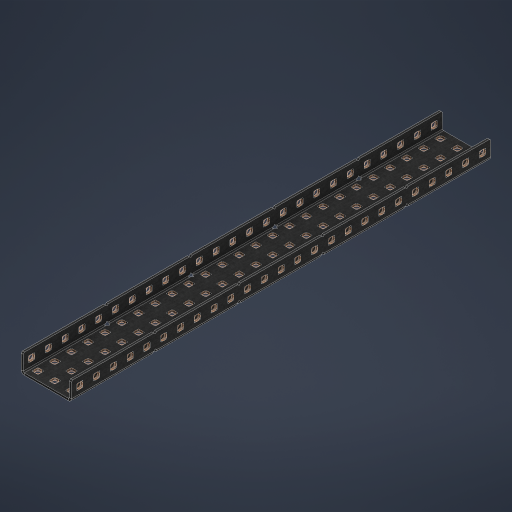
# Autodesk Inventor part: Alu C 1x3x1x35
Saved by Autodesk Inventor 2024 (Build 280153000, 153)
## iProperties
Created: 2022-07-28
Part Number: Alu C 1x3x1x35
Material: Generic
Document SubType Name: Sheet Metal
Designer: ylu12
Density: 1 g/cm^3
Sheet Metal Rule: Default
Appearance: Aluminum
Author: ylu12
Autodesk Inventor part; units mm, degrees
ref_plane "YZ Plane" through (0, 0, 0) normal (1, 0, 0) x (0, 1, 0)
ref_plane "XZ Plane" through (0, 0, 0) normal (0, 1, 0) x (-1, 0, 0)
ref_plane "XY Plane" through (0, 0, 0) normal (0, 0, 1) x (1, 0, 0)
sketch "Sketch1" plane through (0, 0, 0) normal (0, 1, 0) x (-1, 0, 0)
  line L0 (-19.05, 0) -> (19.05, 0)
  line L1 (19.05, 0) -> (19.05, -317.5)
  line L2 (19.05, -317.5) -> (-19.05, -317.5)
  line L3 (-19.05, -317.5) -> (-19.05, 0)
  line L4 (19.05, 0) -> (-19.05, -317.5) construction
  point P0 (0, 0)
  point P1 (0, 0)
  dimension "d0" = 38.1
  dimension "d1" = 317.5
  constraints: 10 end point, 2 parallel, 1 coincident, 1 horizontal, 1 midpoint, 1 perpendicular
  measures "d0" distance of L1.end L2.end
  measures "d1" distance of L0.end L1.end
extrude "Plate1" add sketch "Sketch1" along normal blind 1.5875
sketch "Sketch2" plane through (17.4625, 0, -317.5) normal (1, 0, 0) x (0, 1, 0)
  line L0 (0, 317.5) -> (0, 0)
  line L1 (0, 0) -> (14.2875, 0)
  line L2 (14.2875, 0) -> (14.2875, 317.5)
  line L3 (14.2875, 317.5) -> (0, 317.5)
  constraints: 6 end point, 1 horizontal, 1 perpendicular, 1 vertical
edge flange "Flanges" height 12.7 angle 90 thickness 1.5875 bend radius 0.7937 thickness toward (1, 0, 0) relief straight relief width 1.5875 relief depth 0.7937 corner gap 1.5875 corner form 0 edges at (19.05, 1.5875, -158.75) (-19.05, 1.5875, -158.75) wall of the first edge with corners at (17.4625, 0, 0) (17.4625, 0, -317.5) (17.4625, 14.2875, -317.5) (17.4625, 14.2875, 0)
bend "Bend1"
corner "Corner1"
sketch "Sketch3" plane through (19.05, 2.3812, -317.5) normal (1, 0, 0) x (0, 0, -1)
  line L0 (-312.9534, 7.8677) -> (-309.3466, 7.8677)
  line L1 (-308.8386, 7.3597) -> (-308.8386, 3.7529)
  line L2 (-309.3466, 3.2449) -> (-312.9534, 3.2449)
  line L3 (-313.4614, 3.7529) -> (-313.4614, 7.3597)
  arc A0 (-312.9534, 7.8677) -> (-313.4614, 7.3597) centre (-312.9534, 7.3597) ccw
  arc A1 (-308.8386, 7.3597) -> (-309.3466, 7.8677) centre (-309.3466, 7.3597) ccw
  arc A2 (-309.3466, 3.2449) -> (-308.8386, 3.7529) centre (-309.3466, 3.7529) ccw
  arc A3 (-313.4614, 3.7529) -> (-312.9534, 3.2449) centre (-312.9534, 3.7529) ccw
  line L4 (-317.5, 0) -> (-317.5, 11.9062) construction
  line L5 (-317.5, 11.9062) -> (0, 11.9062) construction
  line L6 (-312.9534, 7.3597) -> (-309.3466, 3.7529) construction
  point P0 (-317.5, -2.3813)
  point P1 (-308.8386, 3.2449)
  point P2 (-313.4614, 3.2449)
  point P3 (-311.15, 5.5563)
  dimension "d16" = 4.6228
  dimension "d17" = 0.508
  dimension "d20" = 6.35
  dimension "d21" = 6.35
  constraints: 10 end point, 8 point on circle, 8 tangent, 4 centre point, 4 point on line, 3 equal radius, 2 parallel, 2 perpendicular, 1 horizontal, 1 midpoint
  measures "d16" distance of point (-308.839, 3.245) point (-313.461, 3.245)
  measures "d17" radius of A0
  measures "d20" distance from line of point (-311.15, 5.556) L4
  measures "d21" distance from line of L5 point (-311.15, 5.556)
extrude "Flange Stamp" cut sketch "Sketch3" against normal blind 1.5875
sketch "Sketch7" plane through (19.05, 2.3812, 0) normal (1, 0, 0) x (0, 0, -1)
  arc A0 (4.5466, 7.8677) -> (4.0386, 7.3597) centre (4.5466, 7.3597) ccw construction
  arc A1 (8.1534, 3.2449) -> (8.6614, 3.7529) centre (8.1534, 3.7529) ccw construction
  circle A2 centre (6.35, 5.5563) radius 2.1844
  line L0 (4.5466, 7.3597) -> (8.1534, 3.7529) construction
  point P0 (0, -2.3813)
  dimension "d46" = 4.3688
  constraints: 2 end point, 1 centre point, 1 midpoint
  measures "d46" diameter of A2
surface extrude "Flange Circle" sketch "Sketch7" against normal up to surface (1.5875 mm away) shown yes curves A2
ref_plane "Flange Pattern Plane" through (19.05, 7.9375, -4.5466) normal (0, 1, 0) x (1, 0, 0)
pattern_sketch "Flange Pattern" of "Flange Circle", "Flange Stamp" from (19.05, 7.9375, -6.35) facing (1, 0, 0) copies at (19.05, 7.9375, -19.05) facing (1, 0, 0) at (19.05, 7.9375, -31.75) facing (1, 0, 0) at (19.05, 7.9375, -44.45) facing (1, 0, 0) at (19.05, 7.9375, -57.15) facing (1, 0, 0) at (19.05, 7.9375, -69.85) facing (1, 0, 0) at (-19.05, 7.9375, -6.35) facing (-1, 0, 0) at (-19.05, 7.9375, -19.05) facing (-1, 0, 0) at (-19.05, 7.9375, -31.75) facing (-1, 0, 0) at (-19.05, 7.9375, -44.45) facing (-1, 0, 0) at (-19.05, 7.9375, -57.15) facing (-1, 0, 0) at (-19.05, 7.9375, -69.85) facing (-1, 0, 0) at (19.05, 7.9375, -82.55) facing (1, 0, 0) at (-19.05, 7.9375, -82.55) facing (-1, 0, 0) at (19.05, 7.9375, -95.25) facing (1, 0, 0) at (-19.05, 7.9375, -95.25) facing (-1, 0, 0) at (19.05, 7.9375, -107.95) facing (1, 0, 0) at (-19.05, 7.9375, -107.95) facing (-1, 0, 0) at (19.05, 7.9375, -120.65) facing (1, 0, 0) at (-19.05, 7.9375, -120.65) facing (-1, 0, 0) at (19.05, 7.9375, -133.35) facing (1, 0, 0) at (-19.05, 7.9375, -133.35) facing (-1, 0, 0) at (19.05, 7.9375, -146.05) facing (1, 0, 0) at (-19.05, 7.9375, -146.05) facing (-1, 0, 0) at (19.05, 7.9375, -158.75) facing (1, 0, 0) at (-19.05, 7.9375, -158.75) facing (-1, 0, 0) at (19.05, 7.9375, -171.45) facing (1, 0, 0) at (-19.05, 7.9375, -171.45) facing (-1, 0, 0) at (19.05, 7.9375, -184.15) facing (1, 0, 0) at (-19.05, 7.9375, -184.15) facing (-1, 0, 0) at (19.05, 7.9375, -196.85) facing (1, 0, 0) at (-19.05, 7.9375, -196.85) facing (-1, 0, 0) at (19.05, 7.9375, -209.55) facing (1, 0, 0) at (-19.05, 7.9375, -209.55) facing (-1, 0, 0) at (19.05, 7.9375, -222.25) facing (1, 0, 0) at (-19.05, 7.9375, -222.25) facing (-1, 0, 0) at (19.05, 7.9375, -234.95) facing (1, 0, 0) at (-19.05, 7.9375, -234.95) facing (-1, 0, 0) at (19.05, 7.9375, -247.65) facing (1, 0, 0) at (-19.05, 7.9375, -247.65) facing (-1, 0, 0) at (19.05, 7.9375, -260.35) facing (1, 0, 0) at (-19.05, 7.9375, -260.35) facing (-1, 0, 0) at (19.05, 7.9375, -273.05) facing (1, 0, 0) at (-19.05, 7.9375, -273.05) facing (-1, 0, 0) at (19.05, 7.9375, -285.75) facing (1, 0, 0) at (-19.05, 7.9375, -285.75) facing (-1, 0, 0) at (19.05, 7.9375, -298.45) facing (1, 0, 0) at (-19.05, 7.9375, -298.45) facing (-1, 0, 0) at (19.05, 7.9375, -311.15) facing (1, 0, 0) at (-19.05, 7.9375, -311.15) facing (-1, 0, 0)
sketch "Sketch8" plane through (0, 0, 0) normal (0, -1, 0) x (1, 0, 0)
  line L0 (16.6687, 0) -> (-16.6687, 0) construction
  line L1 (14.5034, -4.0386) -> (10.8966, -4.0386)
  line L2 (10.3886, -4.5466) -> (10.3886, -8.1534)
  line L3 (10.8966, -8.6614) -> (14.5034, -8.6614)
  line L4 (15.0114, -8.1534) -> (15.0114, -4.5466)
  arc A0 (15.0114, -4.5466) -> (14.5034, -4.0386) centre (14.5034, -4.5466) ccw
  arc A1 (14.5034, -8.6614) -> (15.0114, -8.1534) centre (14.5034, -8.1534) ccw
  arc A2 (10.3886, -8.1534) -> (10.8966, -8.6614) centre (10.8966, -8.1534) ccw
  arc A3 (10.8966, -4.0386) -> (10.3886, -4.5466) centre (10.8966, -4.5466) ccw
  line L5 (14.5034, -4.5466) -> (10.8966, -8.1534) construction
  line L6 (19.05, 0) -> (19.05, -317.5) construction
  point P0 (0, 0)
  point P1 (10.3886, -8.6614)
  point P2 (15.0114, -8.6614)
  point P3 (12.7, -6.35)
  dimension "d49" = 4.6228
  dimension "d50" = 0.508
  dimension "d51" = 6.35
  dimension "d52" = 6.35
  constraints: 10 end point, 8 point on circle, 8 tangent, 4 centre point, 4 point on line, 3 equal radius, 2 parallel, 2 perpendicular, 1 horizontal, 1 midpoint
  measures "d49" distance of point (15.011, -8.661) point (10.389, -8.661)
  measures "d50" radius of A0
  measures "d51" distance from line of L6 point (12.7, -6.35)
  measures "d52" distance from line of L0 point (12.7, -6.35)
extrude "Body Stamp" cut sketch "Sketch8" against normal blind 1.5875
sketch "Sketch9" plane through (0, 0, 0) normal (0, -1, 0) x (1, 0, 0)
  arc A0 (15.0114, -4.5466) -> (14.5034, -4.0386) centre (14.5034, -4.5466) ccw construction
  arc A1 (10.3886, -8.1534) -> (10.8966, -8.6614) centre (10.8966, -8.1534) ccw construction
  line L0 (14.5034, -4.5466) -> (10.8966, -8.1534) construction
  circle A2 centre (12.7, -6.35) radius 2.1844
  point P0 (0, 0)
  dimension "d55" = 4.3688
  constraints: 2 end point, 1 centre point, 1 midpoint
  measures "d55" diameter of A2
surface extrude "Body Circle" sketch "Sketch9" against normal up to surface (1.5875 mm away) shown yes curves A2
pattern_sketch "Body Pattern" of "Body Stamp", "Body Circle" from (12.7, 0, -6.35) copies at (12.7, 0, -19.05) at (12.7, 0, -31.75) at (12.7, 0, -44.45) at (12.7, 0, -57.15) at (12.7, 0, -69.85) at (12.7, 0, -82.55) at (12.7, 0, -95.25) at (12.7, 0, -107.95) at (12.7, 0, -120.65) at (12.7, 0, -133.35) at (12.7, 0, -146.05) at (12.7, 0, -158.75) at (12.7, 0, -171.45) at (12.7, 0, -184.15) at (12.7, 0, -196.85) at (12.7, 0, -209.55) at (12.7, 0, -222.25) at (12.7, 0, -234.95) at (12.7, 0, -247.65) at (12.7, 0, -260.35) at (12.7, 0, -273.05) at (12.7, 0, -285.75) at (12.7, 0, -298.45) at (12.7, 0, -311.15) at (0, 0, -6.35) at (0, 0, -19.05) at (0, 0, -31.75) at (0, 0, -44.45) at (0, 0, -57.15) at (0, 0, -69.85) at (0, 0, -82.55) at (0, 0, -95.25) at (0, 0, -107.95) at (0, 0, -120.65) at (0, 0, -133.35) at (0, 0, -146.05) at (0, 0, -158.75) at (0, 0, -171.45) at (0, 0, -184.15) at (0, 0, -196.85) at (0, 0, -209.55) at (0, 0, -222.25) at (0, 0, -234.95) at (0, 0, -247.65) at (0, 0, -260.35) at (0, 0, -273.05) at (0, 0, -285.75) at (0, 0, -298.45) at (0, 0, -311.15) at (-12.7, 0, -6.35) at (-12.7, 0, -19.05) at (-12.7, 0, -31.75) at (-12.7, 0, -44.45) at (-12.7, 0, -57.15) at (-12.7, 0, -69.85) at (-12.7, 0, -82.55) at (-12.7, 0, -95.25) at (-12.7, 0, -107.95) at (-12.7, 0, -120.65) at (-12.7, 0, -133.35) at (-12.7, 0, -146.05) at (-12.7, 0, -158.75) at (-12.7, 0, -171.45) at (-12.7, 0, -184.15) at (-12.7, 0, -196.85) at (-12.7, 0, -209.55) at (-12.7, 0, -222.25) at (-12.7, 0, -234.95) at (-12.7, 0, -247.65) at (-12.7, 0, -260.35) at (-12.7, 0, -273.05) at (-12.7, 0, -285.75) at (-12.7, 0, -298.45) at (-12.7, 0, -311.15)
sketch "Arc Length" plane through (17.4625, 2.3812, 0) normal (0, 0, 1) x (1, 0, 0)
  line L0 (0, 0) -> (1.5875, 0) construction
  arc A0 (-0.7937, -0.7937) -> (0, 0) centre (-0.7937, 0) ccw construction
  line L1 (-0.7937, -2.3812) -> (-0.7937, -0.7937) construction
  arc A1 (-0.7937, -2.3812) -> (1.5875, 0) centre (-0.7937, 0) ccw construction
  point P0 (-17.4625, -2.3812)
  dimension "d85" = 3.7405
  dimension "d92" = 1.2468
sketch "Sketch13" plane through (19.05, 14.2875, 0) normal (1, 0, 0) x (0, 0, -1)
  line L0 (0, 0) -> (317.5, 0) construction
  line L1 (62.4078, 0) -> (63.4238, -1.016)
  line L2 (63.4238, -1.016) -> (64.4398, 0)
  line L3 (62.4078, 0) -> (64.4398, 0)
  line L4 (317.5, -11.9062) -> (0, -11.9062) construction
  line L5 (63.4238, -10.8903) -> (61.161, -13.1531)
  line L6 (61.161, -13.1531) -> (63.4238, -15.4159)
  line L7 (63.4238, -15.4159) -> (65.6866, -13.1531)
  line L8 (65.6866, -13.1531) -> (63.4238, -10.8903)
  line L9 (63.4238, -10.8903) -> (63.4238, -15.4159) construction
  line L10 (63.4238, -1.016) -> (63.4238, -10.8903) construction
  line L11 (0, -11.9062) -> (317.5, -11.9062) construction
  point P0 (0, -14.2875)
  dimension "d86" = 4.5256
  dimension "d88" = 1.016
  dimension "d91" = 1.016
  dimension "d102" = 63.4238
  constraints: 19 end point, 6 perpendicular, 2 point on line, 2 vertical, 1 collinear
  measures "d86" distance of L5.start L6.end
  measures "d88" distance from line of L0 L1.end
  measures "d91" distance from line of L5.start L11
  measures "d102" distance from line of L0.start L10
cut across bends "Notch" sketch "Sketch13" k factor 0.44
mirror "Notch Mirror" about plane through (0, 0, 0) normal (1, 0, 0) of "Notch"
pattern_linear "Notch Pattern" count 4 spacing 63.5 along (0, 0, -1) of "Notch", "Notch Mirror"
chamfer "End Chamfer" distance 1.016 angle 45 4 edges at (-18.2562, 14.2875, 0) (18.2562, 14.2875, 0) (-18.2562, 14.2875, -317.5) (18.2563, 14.2875, -317.5)
sketch "Sketch14" plane through (-19.05, 2.3813, 127) normal (1, 0, 0) x (0, 0, -1)
  line L0 (127, 11.9063) -> (444.5, 11.9063) construction
  line L1 (127, 0) -> (127, 11.9063) construction
  line L2 (127, -2.3813) -> (444.5, -2.3813) construction
  line L3 (127, 11.9063) -> (444.5, 11.9063)
  line L4 (444.5, 11.9063) -> (444.5, -2.3813)
  line L5 (444.5, -2.3813) -> (127, -2.3813)
  line L6 (127, -2.3813) -> (127, 11.9063)
  point P0 (127, -2.3812)
  point P1 (382.0521, -1.9844)
  constraints: 8 end point, 2 collinear, 2 parallel, 1 horizontal, 1 perpendicular, 1 other
extrude "Half Cut" [suppressed]
sketch "Flange Pattern Sketch" plane through (19.05, 7.9375, -4.5466) normal (0, 1, 0) x (1, 0, 0)
  line L0 (0, 3.6068) -> (0, 0) construction
  line L1 (-45.8186, -4.5466) -> (8.2118, -4.5466) construction
  line L2 (0, 0) -> (-1.5875, 0) construction
  point P0 (-19.05, -4.5466)
  point P1 (0, 1.8034)
  point P2 (0, 14.5034)
  point P3 (0, 27.2034)
  point P4 (0, 39.9034)
  point P5 (0, 52.6034)
  point P6 (0, 65.3034)
  point P7 (-38.1, 1.8034)
  point P8 (-38.1, 14.5034)
  point P9 (-38.1, 27.2034)
  point P10 (-38.1, 39.9034)
  point P11 (-38.1, 52.6034)
  point P12 (-38.1, 65.3034)
  point P13 (0, 78.0034)
  point P14 (-38.1, 78.0034)
  point P15 (0, 90.7034)
  point P16 (-38.1, 90.7034)
  point P17 (0, 103.4034)
  point P18 (-38.1, 103.4034)
  point P19 (0, 116.1034)
  point P20 (-38.1, 116.1034)
  point P21 (0, 128.8034)
  point P22 (-38.1, 128.8034)
  point P23 (0, 141.5034)
  point P24 (-38.1, 141.5034)
  point P25 (0, 154.2034)
  point P26 (-38.1, 154.2034)
  point P27 (0, 166.9034)
  point P28 (-38.1, 166.9034)
  point P29 (0, 179.6034)
  point P30 (-38.1, 179.6034)
  point P31 (0, 192.3034)
  point P32 (-38.1, 192.3034)
  point P33 (0, 205.0034)
  point P34 (-38.1, 205.0034)
  point P35 (0, 217.7034)
  point P36 (-38.1, 217.7034)
  point P37 (0, 230.4034)
  point P38 (-38.1, 230.4034)
  point P39 (0, 243.1034)
  point P40 (-38.1, 243.1034)
  point P41 (0, 255.8034)
  point P42 (-38.1, 255.8034)
  point P43 (0, 268.5034)
  point P44 (-38.1, 268.5034)
  point P45 (0, 281.2034)
  point P46 (-38.1, 281.2034)
  point P47 (0, 293.9034)
  point P48 (-38.1, 293.9034)
  point P49 (0, 306.6034)
  point P50 (-38.1, 306.6034)
  dimension "d131" = 38.1
  dimension "d134" = 12.7
  constraints: 1 horizontal, 1 midpoint, 1 vertical, 49 other
  measures "d134" distance of point (0, 1.803) point (0, 14.503)
sketch "Body Pattern Sketch" plane through (0, 0, 0) normal (0, -1, 0) x (1, 0, 0)
  line L0 (16.6687, 0) -> (-16.6687, 0) construction
  line L1 (19.05, 0) -> (19.05, -317.5) construction
  circle A0 centre (12.7, -6.35) radius 2.1844 construction
  point P0 (0, 0)
  point P1 (12.7, -19.05)
  point P2 (12.7, -31.75)
  point P3 (12.7, -44.45)
  point P4 (12.7, -57.15)
  point P5 (12.7, -69.85)
  point P6 (12.7, -82.55)
  point P7 (12.7, -95.25)
  point P8 (12.7, -107.95)
  point P9 (12.7, -120.65)
  point P10 (12.7, -133.35)
  point P11 (12.7, -146.05)
  point P12 (12.7, -158.75)
  point P13 (12.7, -171.45)
  point P14 (12.7, -184.15)
  point P15 (12.7, -196.85)
  point P16 (12.7, -209.55)
  point P17 (12.7, -222.25)
  point P18 (12.7, -234.95)
  point P19 (12.7, -247.65)
  point P20 (12.7, -260.35)
  point P21 (12.7, -273.05)
  point P22 (12.7, -285.75)
  point P23 (12.7, -298.45)
  point P24 (12.7, -311.15)
  point P25 (0, -6.35)
  point P26 (0, -19.05)
  point P27 (0, -31.75)
  point P28 (0, -44.45)
  point P29 (0, -57.15)
  point P30 (0, -69.85)
  point P31 (0, -82.55)
  point P32 (0, -95.25)
  point P33 (0, -107.95)
  point P34 (0, -120.65)
  point P35 (0, -133.35)
  point P36 (0, -146.05)
  point P37 (0, -158.75)
  point P38 (0, -171.45)
  point P39 (0, -184.15)
  point P40 (0, -196.85)
  point P41 (0, -209.55)
  point P42 (0, -222.25)
  point P43 (0, -234.95)
  point P44 (0, -247.65)
  point P45 (0, -260.35)
  point P46 (0, -273.05)
  point P47 (0, -285.75)
  point P48 (0, -298.45)
  point P49 (0, -311.15)
  point P50 (-12.7, -6.35)
  point P51 (-12.7, -19.05)
  point P52 (-12.7, -31.75)
  point P53 (-12.7, -44.45)
  point P54 (-12.7, -57.15)
  point P55 (-12.7, -69.85)
  point P56 (-12.7, -82.55)
  point P57 (-12.7, -95.25)
  point P58 (-12.7, -107.95)
  point P59 (-12.7, -120.65)
  point P60 (-12.7, -133.35)
  point P61 (-12.7, -146.05)
  point P62 (-12.7, -158.75)
  point P63 (-12.7, -171.45)
  point P64 (-12.7, -184.15)
  point P65 (-12.7, -196.85)
  point P66 (-12.7, -209.55)
  point P67 (-12.7, -222.25)
  point P68 (-12.7, -234.95)
  point P69 (-12.7, -247.65)
  point P70 (-12.7, -260.35)
  point P71 (-12.7, -273.05)
  point P72 (-12.7, -285.75)
  point P73 (-12.7, -298.45)
  point P74 (-12.7, -311.15)
  dimension "d62" = 12.7
  dimension "d65" = 12.7
  dimension "d139" = 12.7
  constraints: 1 coincident, 1 horizontal, 1 vertical, 74 other
  measures "d139" distance of point (12.7, -19.05) point (12.7, -6.35)
equation "\"d18\" = Thickness"
equation "\"d53\" = Thickness"
equation "\"d89\" = Thickness"
equation "\"d1\" = 12.7 * Length"
equation "\"d2\" = Thickness"
equation "\"d3\" = BendReliefWidth"
equation "\"d4\" = BendReliefDepth"
equation "\"d5\" = MinimumRemnant"
equation "\"d6\" = TransitionRadius"
equation "\"d10\" = CornerReliefSize"
equation "\"d11\" = GapSize"
equation "\"d12\" = JacobiRadiusSize"
equation "\"BendRadius\" = Thickness"
equation "\"BendReliefWidth\" = Thickness"
equation "\"BendReliefDepth\" = 0.5 * Thickness"
equation "\"CornerReliefSize\" = 4 * Thickness"
equation "\"MinimumRemnant\" = 2 * Thickness"
equation "\"TransitionRadius\" = BendRadius"
equation "\"JacobiRadiusSize\" = BendRadius"
equation "\"GapSize\" = Thickness"
equation "\"Thickness\" = 1.5875"
equation "\"Length\" = 25"
body "Solid1"
body "Srf1"
body "Srf2"
body "Srf91"
body "Srf92"
body "Srf856"
body "Srf1310"
body "Srf1311"
body "Srf1312"
body "Srf1376"
body "Srf1377"
body "Srf1728"
body "Srf1755"
body "Srf1878"
body "Srf1879"
body "Srf1880"
body "Srf1881"
body "Srf1882"
body "Srf1883"
body "Srf1884"
body "Srf1885"
body "Srf1886"
body "Srf1887"
body "Srf1888"
body "Srf1889"
body "Srf1890"
body "Srf1891"
body "Srf1892"
body "Srf1893"
body "Srf1894"
body "Srf1895"
body "Srf1896"
body "Srf1897"
body "Srf1898"
body "Srf1899"
body "Srf1900"
body "Srf1901"
body "Srf1902"
body "Srf1903"
body "Srf1904"
body "Srf1905"
body "Srf1906"
body "Srf1907"
body "Srf1908"
body "Srf1909"
body "Srf1910"
body "Srf1911"
body "Srf1912"
body "Srf1913"
body "Srf1914"
body "Srf1915"
body "Srf1916"
body "Srf1917"
body "Srf1918"
body "Srf1919"
body "Srf1920"
body "Srf1921"
body "Srf1942"
body "Srf1943"
body "Srf1944"
body "Srf1945"
body "Srf1946"
body "Srf1947"
body "Srf1948"
body "Srf1949"
body "Srf1950"
body "Srf1951"
body "Srf1952"
body "Srf1953"
body "Srf1954"
body "Srf1955"
body "Srf1956"
body "Srf1957"
body "Srf1958"
body "Srf1959"
body "Srf1960"
body "Srf1961"
body "Srf1962"
body "Srf1963"
body "Srf1964"
body "Srf1965"
body "Srf1966"
body "Srf1967"
body "Srf1968"
body "Srf1969"
body "Srf1970"
body "Srf1971"
body "Srf1972"
body "Srf1973"
body "Srf1974"
body "Srf1975"
body "Srf1976"
body "Srf1977"
body "Srf1978"
body "Srf1979"
body "Srf1980"
body "Srf1981"
body "Srf1982"
body "Srf1983"
body "Srf1984"
body "Srf1985"
body "Srf1986"
body "Srf1987"
body "Srf1988"
body "Srf1989"
body "Srf1990"
body "Srf1991"
body "Srf1992"
body "Srf1993"
body "Srf1994"
body "Srf1995"
body "Srf1996"
body "Srf1997"
body "Srf1998"
body "Srf1999"
body "Srf2000"
body "Srf2001"
body "Srf2002"
body "Srf2003"
body "Srf2004"
body "Srf2005"
body "Srf2006"
body "Srf2007" dims "d2" = 1.5875 (= Thickness), "d10" = 6.35 (= CornerReliefSize)
body "Srf2008"
body "Srf2009"
body "Srf2010"
